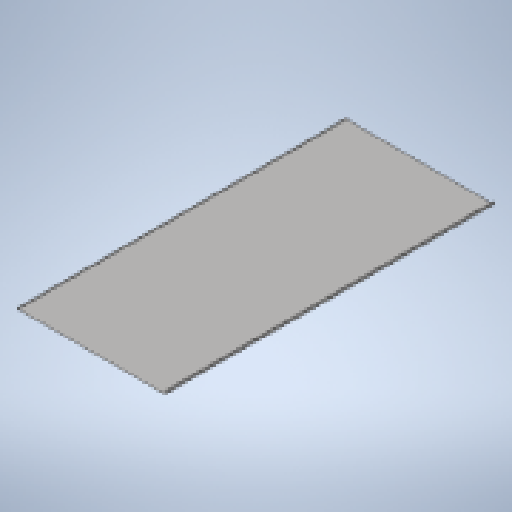
# Autodesk Inventor part: MSC 0102 sheet gills
Saved by Autodesk Inventor 2025 (Build 290162010, 162A)
## iProperties
Created: 2024-06-15
Part Number: MSC 0102 sheet gills
Material: Stainless Steel
Document SubType Name: Sheet Metal
Designer: admin
Stock Number: МОО 0101 лист жабра
Mass: 8000 g
Surface Area: 40030 cm^2
Volume: 1000 cm^3
Density: 8 g/cm^3
Sheet Metal Rule: Default_mm
Appearance: Default
Author: pokla
Autodesk Inventor part; units mm, degrees
ref_plane "YZ Plane" through (0, 0, 0) normal (1, 0, 0) x (0, 1, 0)
ref_plane "XZ Plane" through (0, 0, 0) normal (0, 1, 0) x (-1, 0, 0)
ref_plane "XY Plane" through (0, 0, 0) normal (0, 0, 1) x (1, 0, 0)
sketch "Sketch6" plane through (0, 0, 0) normal (0, 1, 0) x (-1, 0, 0)
  line L0 (454, -1000) -> (-454, -1000)
  line L1 (-454, -1000) -> (-454, 1000)
  line L2 (-454, 1000) -> (454, 1000)
  line L3 (454, 1000) -> (454, -1000)
  line L4 (454, -1000) -> (-454, 1000) construction
  line L5 (-454, -1000) -> (454, 1000) construction
  point P0 (0, 0)
  dimension "d52" = 908
  dimension "d53" = 2000
  measures "d52" distance of L1.end L2.end
  measures "d53" distance of L0.end L1.end
extrude "Plate2" add sketch "Sketch6" along normal blind 0.5
sketch "Sketch10" plane through (-453.5, 0, 1000) normal (-1, 0, 0) x (0, -1, 0)
  line L0 (0, -2000) -> (0, 0)
  line L1 (0, 0) -> (-10, 0)
  line L2 (-10, 0) -> (-10, -2000)
  line L3 (-10, -2000) -> (0, -2000)
  constraints: 6 end point, 1 horizontal, 1 perpendicular, 1 vertical
edge flange "Flange1" height 10 angle 90 thickness 0.5 bend radius 0.5 thickness toward (-1, 0, 0) relief straight relief width 0.5 relief depth 0.25 corner gap 0.5 corner form 0 edges at (-454, 0.5, 0) (454, 0.5, 0) wall of the first edge with corners at (-453.5, 0, -1000) (-453.5, 0, 1000) (-453.5, 10, 1000) (-453.5, 10, -1000)
bend "Bend2"
corner "Corner2"
sketch "Sketch11" plane through (454, 9.5, -1000) normal (0, 1, 0) x (-1, 0, 0)
  line L0 (0, 2000) -> (0, 0)
  line L1 (0, 0) -> (10, 0)
  line L2 (10, 0) -> (10, 2000)
  line L3 (10, 2000) -> (0, 2000)
  constraints: 6 end point, 1 horizontal, 1 perpendicular, 1 vertical
edge flange "Flange2" height 10 angle 90 thickness 0.5 bend radius 0.5 thickness toward (0, 1, 0) relief straight relief width 0.5 relief depth 0.25 corner gap 0.5 corner form 0 edges at (453.5, 10, 0) (-453.5, 10, 0) wall of the first edge with corners at (454, 9.5, 1000) (454, 9.5, -1000) (444, 9.5, -1000) (444, 9.5, 1000)
bend "Bend3"
corner "Corner3"
equation "\"d53\" = ЖАБРЫ_базовая_длина_дл_лист"
equation "\"d54\" = Thickness"
equation "\"d74\" = BendReliefWidth"
equation "\"d75\" = BendReliefDepth"
equation "\"d76\" = MinimumRemnant"
equation "\"d77\" = TransitionRadius"
equation "\"d80\" = BendRadius"
equation "\"d81\" = CornerReliefSize"
equation "\"d82\" = GapSize"
equation "\"d83\" = JacobiRadiusSize"
equation "\"d84\" = BendReliefWidth"
equation "\"d85\" = BendReliefDepth"
equation "\"d86\" = MinimumRemnant"
equation "\"d87\" = TransitionRadius"
equation "\"d90\" = BendRadius"
equation "\"d91\" = CornerReliefSize"
equation "\"d92\" = GapSize"
equation "\"d93\" = JacobiRadiusSize"
equation "\"BendRadius\" = Thickness"
equation "\"BendReliefWidth\" = Thickness"
equation "\"BendReliefDepth\" = 0.5 * Thickness"
equation "\"CornerReliefSize\" = 4 * Thickness"
equation "\"MinimumRemnant\" = 2 * Thickness"
equation "\"TransitionRadius\" = BendRadius"
equation "\"JacobiRadiusSize\" = BendRadius"
equation "\"GapSize\" = Thickness"
equation "\"ЖАБРЫ_базовая_длина_дл_лист\" = 2000"
equation "\"Thickness\" = 0.5"
body "Solid2"
